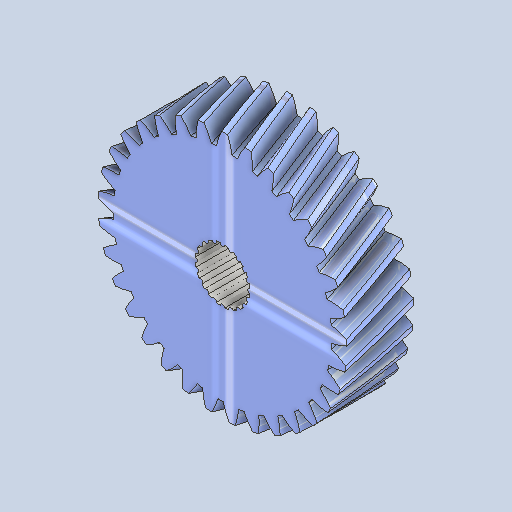
# Autodesk Inventor part: Spur Gear1
Saved by Autodesk Inventor 2025.1 (Build 291241020, 241B)
## iProperties
CustomPartVersion: 1
Created: 2023-08-01
Part Number: Spur Gear1
Material: Steel
Document SubType Name: Modeling
Designer: t205b
Categories: <?xml version="1.0" encoding="UTF-16"?> <MemberInstance><Categories><FamilyTemplate><FamilyTemplateParameter ValueType="xs:double" Id="1" ObjectReferenceKey="da_z" ObjectType="kUserParameterObject"/><FamilyTemplateParameter ValueType="xs:double" Id="2" ObjectReferenceKey="da_b" ObjectType="kUserParameterObject"/><FamilyTemplateParameter ValueType="xs:double" Id="3" ObjectReferenceKey="da_beta" ObjectType="kUserParameterObject"/><FamilyTemplateParameter ValueType="xs:double" Id="4" ObjectReferenceKey="da_da" ObjectType="kUserParameterObject"/><FamilyTemplateParameter ValueType="xs:double" Id="5" ObjectReferenceKey="da_aw" ObjectType="kUserParameterObject"/><FamilyTemplateParameter ValueType="xs:string" Id="6" ObjectReferenceKey="EAIAABAAAACIAQAAAAAAAIAAAAAAAAAA" ObjectType="83910656" SubObjectId="SurfaceGeometry"/></FamilyTemplate><ParamToTemplateMap><ParamToTemplate CategoryParameter="//CategoryParameter[@InternalName='046C89C9-8512-4d59-83FE-43B91F4F132A']" TemplateParameter="1"/><ParamToTemplate CategoryParameter="//CategoryParameter[@InternalName='2552DF32-E462-4b46-AEBF-C6C7768E72AC']" TemplateParameter="2"/><ParamToTemplate CategoryParameter="//CategoryParameter[@InternalName='C9EE641D-15FC-4fae-A226-E94C4372FDD7']" TemplateParameter="3"/><ParamToTemplate><ParamToTemplate CategoryParameter="//CategoryParameter[@InternalName='00B6519A-459B-49c7-AD84-2E56D39A5744']" ConstantValue="0.000000"/></ParamToTemplate><ParamToTemplate><ParamToTemplate CategoryParameter="//CategoryParameter[@InternalName='04B31F0E-C7A6-4894-AA32-9629BEFACF47']" ConstantValue="1.000000"/></ParamToTemplate><ParamToTemplate><ParamToTemplate CategoryParameter="//CategoryParameter[@InternalName='43CBEC2E-7847-49e7-A936-2F7889FCB2D9']" ConstantValue="0.250000"/></ParamToTemplate><ParamToTemplate><ParamToTemplate CategoryParameter="//CategoryParameter[@InternalName='B1EFC894-105D-4ebd-86BF-FA20ED196853']" ConstantValue="0.350000"/></ParamToTemplate><ParamToTemplate><ParamToTemplate CategoryParameter="//CategoryParameter[@InternalName='51175063-3D10-4879-93E8-6246FE8B403D']" ConstantValue="2060000000.000000"/></ParamToTemplate><ParamToTemplate><ParamToTemplate CategoryParameter="//CategoryParameter[@InternalName='A3A52E27-4454-46a9-B0BD-C932399B70AF']" ConstantValue="0.300000"/></ParamToTemplate><ParamToTemplate><ParamToTemplate CategoryParameter="//CategoryParameter[@InternalName='91B76062-C214-41d9-B1B9-14D2AB99603D']" ConstantValue="0.150000"/></ParamToTemplate><ParamToTemplate><ParamToTemplate CategoryParameter="//CategoryParameter[@InternalName='374E806E-8B8A-4dda-A9AA-1039D6500AD2']" ConstantValue="6.666667"/></ParamToTemplate><ParamToTemplate><ParamToTemplate CategoryParameter="//CategoryParameter[@InternalName='2D373A89-B862-43d6-8D0B-0CBF12AB9F6C']" ConstantValue="0.349066"/></ParamToTemplate><ParamToTemplate CategoryParameter="//CategoryParameter[@InternalName='37777632-D6A2-4fac-9D53-DB8ACD95C989']" TemplateParameter="4"/><ParamToTemplate CategoryParameter="//CategoryParameter[@InternalName='FD1017F1-B727-4f7e-9707-0F86F1FF9423']" TemplateParameter="5"/><ParamToTemplate><ParamToTemplate CategoryParameter="//CategoryParameter[@InternalName='9E1B4470-B2D3-4ff1-B813-535BB4CDF51A']" ConstantValue="3520000.000000"/></ParamToTemplate><ParamToTemplate><ParamToTemplate CategoryParameter="//CategoryParameter[@InternalName='F8452263-BFF6-458c-9FB1-07C4B99E95CD']" ConstantValue="11400000.000000"/></ParamToTemplate><ParamToTemplate><ParamToTemplate CategoryParameter="//CategoryParameter[@InternalName='3E3BB259-FD49-497f-8171-6EBC954A3479']" ConstantValue="2.000000"/></ParamToTemplate><ParamToTemplate CategoryParameter="//CategoryParameter[@InternalName='27C3BAF2-7550-4e4b-AE2C-0DB134B7D9B7']" TemplateParameter="6"/></ParamToTemplateMap><Category DisplayName="Gear" InternalName="DC85795E-93AB-48d5-8EEE-5A27447B64BD" Mnemonic="Gear"><CategoryParameter DisplayName="z" InternalName="046C89C9-8512-4d59-83FE-43B91F4F132A" Mnemonic="z"/><CategoryParameter DisplayName="b" InternalName="2552DF32-E462-4b46-AEBF-C6C7768E72AC" Mnemonic="b"/><CategoryParameter DisplayName="||b|" InternalName="C9EE641D-15FC-4fae-A226-E94C4372FDD7" Mnemonic="beta"/><CategoryParameter DisplayName="x" InternalName="00B6519A-459B-49c7-AD84-2E56D39A5744" Mnemonic="x"/><CategoryParameter DisplayName="a*" InternalName="04B31F0E-C7A6-4894-AA32-9629BEFACF47" Mnemonic="a"/><CategoryParameter DisplayName="c*" InternalName="43CBEC2E-7847-49e7-A936-2F7889FCB2D9" Mnemonic="c"/><CategoryParameter DisplayName="r|.f|*" InternalName="B1EFC894-105D-4ebd-86BF-FA20ED196853" Mnemonic="rf"/><CategoryParameter DisplayName="E" InternalName="51175063-3D10-4879-93E8-6246FE8B403D" Mnemonic="E"/><CategoryParameter DisplayName="||m|" InternalName="A3A52E27-4454-46a9-B0BD-C932399B70AF" Mnemonic="mi"/><Category DisplayName="SpurGear" InternalName="26C5A22E-A91E-4dfd-A3B3-23CCAFAE1764" Mnemonic="SpurGear"><CategoryParameter DisplayName="m" InternalName="91B76062-C214-41d9-B1B9-14D2AB99603D" Mnemonic="m"/><CategoryParameter DisplayName="P" InternalName="374E806E-8B8A-4dda-A9AA-1039D6500AD2" Mnemonic="PP"/><CategoryParameter DisplayName="||a|" InternalName="2D373A89-B862-43d6-8D0B-0CBF12AB9F6C" Mnemonic="alpha"/><CategoryParameter DisplayName="d|.a|" InternalName="37777632-D6A2-4fac-9D53-DB8ACD95C989" Mnemonic="da"/><CategoryParameter DisplayName="a|.w|" InternalName="FD1017F1-B727-4f7e-9707-0F86F1FF9423" Mnemonic="aw"/><CategoryParameter DisplayName="||s||.Flim|" InternalName="9E1B4470-B2D3-4ff1-B813-535BB4CDF51A" Mnemonic="sFlim"/><CategoryParameter DisplayName="||s||.Hlim|" InternalName="F8452263-BFF6-458c-9FB1-07C4B99E95CD" Mnemonic="sHlim"/><CategoryParameter DisplayName="type" InternalName="3E3BB259-FD49-497f-8171-6EBC954A3479" Mnemonic="type"/><CategoryParameter DisplayName="PitchDiameter" InternalName="27C3BAF2-7550-4e4b-AE2C-0DB134B7D9B7" Mnemonic="IDS_PITCHDIAM"/></Category></Category></Categories></MemberInstance>
Density: 1 g/cm^3
Appearance: Steel
Author: t205b
Autodesk Inventor part; units mm, degrees
sketch "Sketch1" plane through (0, 0, 0) normal (0, 0, 1) x (1, 0, 0)
  circle A0 centre (0, 0) radius 27.8382
  dimension "d0" = 55.6764
  constraints: 1 centre point
  measures "d0" diameter of A0
extrude "Extrusion1" add sketch "Sketch1" along normal blind 15
ref_plane "Work Plane2" through (0, 0, 7.5) normal (0, 0, 1) x (1, 0, 0)
sketch "Sketch2" plane through (0, 0, 0) normal (0, 0, -1) x (-1, 0, 0)
  circle A0 centre (0, 0) radius 27.8382 projected
  circle A1 centre (0, 0) radius 26.3384
  dimension "d3" = 52.6768
  constraints: 1 centre point, 1 coincident
  measures "d3" diameter of A1
surface extrude "Pitch Diameter" sketch "Sketch2" against normal through all shown no curves A1
ref_plane "Work Plane8" through (0, 0, 0) normal (0.9954719, 0.095056, 0) x (0, 0, 1)
ref_plane "Work Plane9" through (0, 0, 0) normal (1, 0, 0) x (0, 1, 0)
spur gear teeth "Spur Gear" teeth 33 pitch diameter 52.6768 tip diameter 55.6764 root diameter 48.9268 face width 15 helix angle 20 hand left start plane through (0, 0, 0) normal (0, 0, -1) x (-1, 0, 0)
sketch "Sketch3" plane through (0, 0, 15) normal (0, 0, 1) x (1, 0, 0)
  circle A0 centre (0, 0) radius 6.1085
  arc A1 (-0.5143, 6.0868) -> (0.5143, 6.0868) centre (0, 6.1135) ccw
  line L0 (0, 6.1135) -> (0.5143, 6.0868) construction
  line L1 (0, 6.1135) -> (-0.5143, 6.0868) construction
  arc A2 (-2.3701, 5.63) -> (-1.3918, 5.9478) centre (-1.8892, 5.8143) ccw
  arc A3 (-3.9938, 4.622) -> (-3.1617, 5.2266) centre (-3.5934, 4.9459) ccw
  arc A4 (-5.2266, 3.1617) -> (-4.622, 3.9938) centre (-4.9459, 3.5934) ccw
  arc A5 (-5.9478, 1.3918) -> (-5.63, 2.3701) centre (-5.8143, 1.8892) ccw
  arc A6 (-6.0868, -0.5143) -> (-6.0868, 0.5143) centre (-6.1135, 0) ccw
  arc A7 (-5.63, -2.3701) -> (-5.9478, -1.3918) centre (-5.8143, -1.8892) ccw
  arc A8 (-4.622, -3.9938) -> (-5.2266, -3.1617) centre (-4.9459, -3.5934) ccw
  arc A9 (-3.1617, -5.2266) -> (-3.9938, -4.622) centre (-3.5934, -4.9459) ccw
  arc A10 (-1.3918, -5.9478) -> (-2.3701, -5.63) centre (-1.8892, -5.8143) ccw
  arc A11 (0.5143, -6.0868) -> (-0.5143, -6.0868) centre (0, -6.1135) ccw
  arc A12 (2.3701, -5.63) -> (1.3918, -5.9478) centre (1.8892, -5.8143) ccw
  arc A13 (3.9938, -4.622) -> (3.1617, -5.2266) centre (3.5934, -4.9459) ccw
  arc A14 (5.2266, -3.1617) -> (4.622, -3.9938) centre (4.9459, -3.5934) ccw
  arc A15 (5.9478, -1.3918) -> (5.63, -2.3701) centre (5.8143, -1.8892) ccw
  arc A16 (6.0868, 0.5143) -> (6.0868, -0.5143) centre (6.1135, 0) ccw
  arc A17 (5.63, 2.3701) -> (5.9478, 1.3918) centre (5.8143, 1.8892) ccw
  arc A18 (4.622, 3.9938) -> (5.2266, 3.1617) centre (4.9459, 3.5934) ccw
  arc A19 (3.1617, 5.2266) -> (3.9938, 4.622) centre (3.5934, 4.9459) ccw
  arc A20 (1.3918, 5.9478) -> (2.3701, 5.63) centre (1.8892, 5.8143) ccw
  point P0 (1.3918, 5.9478)
  point P1 (-1.3918, 5.9478)
  point P2 (-2.3701, 5.63)
  point P3 (-3.1617, 5.2266)
  point P4 (-3.9938, 4.622)
  point P5 (-5.2266, 3.1617)
  point P6 (-5.63, 2.3701)
  point P7 (-5.9478, 1.3918)
  point P8 (-6.0868, 0.5143)
  point P9 (-6.0868, -0.5143)
  point P10 (-5.9478, -1.3918)
  point P11 (-5.63, -2.3701)
  point P12 (-5.2266, -3.1617)
  point P13 (-3.9938, -4.622)
  point P14 (-2.3701, -5.63)
  point P15 (-1.3918, -5.9478)
  point P16 (-0.5143, -6.0868)
  point P17 (0.5143, -6.0868)
  point P18 (1.3918, -5.9478)
  point P19 (2.3701, -5.63)
  point P20 (3.1617, -5.2266)
  point P21 (4.622, -3.9938)
  point P22 (6.0868, -0.5143)
  point P23 (6.0868, 0.5143)
  point P24 (5.9478, 1.3918)
  point P25 (5.63, 2.3701)
  point P26 (3.9938, 4.622)
  point P27 (3.1617, 5.2266)
  dimension "d49" = 12.217
  dimension "d53" = 0.515
  dimension "d54" = 6.1135
  dimension "d57" = 360
  constraints: 40 point on circle, 20 centre point, 4 end point, 1 coincident, 1 vertical alignment, 85 other
  measures "d53" radius of A1
  measures "d54" distance of L0.start point (0, 0)
extrude "Extrusion2" cut sketch "Sketch3" against normal through all contours A16 A0 A15 A14 A13 A12 A11 A10 A9 A8 A7 A6 A5 A4 A3 A2 A1 A20 A19 A18 A17
equation "\"d0\" = da_da"
equation "\"d1\" = da_b"
equation "\"d3\" = da_d"
equation "\"d16\" = da_aw"
equation "\"d43\" = da_aw"
equation "\"d46\" = da_aw"
equation "\"da_da\" = 55.676444"
equation "\"da_b\" = 15"
equation "\"da_d\" = 52.6768"
equation "\"da_aw\" = 63.909111"
body "Solid1"
body "Srf1"
